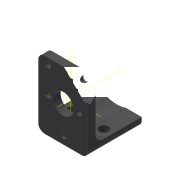
# Autodesk Inventor part: empty
Saved by Autodesk Inventor 2014 (Build 180170000, 170)
## iProperties
Created: 2015-04-13
Part Number: empty
Material: Generic
Document SubType Name: Modeling
Designer: Martin
Density: 1 g/cm^3
Appearance: Default
Author: Martin
Autodesk Inventor part; units mm, degrees
ref_plane "YZ Plane" through (0, 0, 0) normal (1, 0, 0) x (0, 1, 0)
ref_plane "XZ Plane" through (0, 0, 0) normal (0, 1, 0) x (-1, 0, 0)
ref_plane "XY Plane" through (0, 0, 0) normal (0, 0, 1) x (1, 0, 0)
sketch "sk_main" plane through (0, 0, 0) normal (1, 0, 0) x (0, 1, 0)
  line L0 (-8, 0) -> (30.5, 0) projected
  line L1 (0, -15.9) -> (0, 14.9) projected
  line L2 (25, -7.5) -> (0, -7.5)
  line L3 (0, -7.5) -> (0, 9)
  line L4 (25, -11.5) -> (-2.5, -11.5)
  line L5 (-2.5, -11.5) -> (-2.5, 10.5)
  line L6 (0, 10.5) -> (0, -11.5)
  line L7 (25, -7.5) -> (25, -11.5)
  line L8 (-2.5, 10.5) -> (0, 10.5)
  point P0 (0, 0)
  dimension "d5" = 2.5
  dimension "d35" = 25
  dimension "d37" = 4
  dimension "d38" = 18
  dimension "d58" = 10.5
  constraints: 14 end point, 4 perpendicular, 3 point on line, 1 collinear, 1 horizontal, 1 parallel
  measures "d5" distance between parallel lines of L3 L5
  measures "d35" distance of L2.start L2.end
  measures "d37" distance of L2.start L4.start
  measures "d38" distance between parallel lines of L2 L8
  measures "d58" distance between parallel lines of L8 L0
extrude "ext_main_back" [suppressed]
extrude "ext_main_front" add sketch "sk_main" along normal mid plane 12.15 contours L5 L8 L1 L0 | L0 L1 L4 L5
sketch "sk_front" plane through (0, 0, 0) normal (0, 1, 0) x (-1, 0, 0)
  line L0 (0, -22.55) -> (0, 16.3) projected
  line L1 (12.1092, 0) -> (-12.1092, 0) projected
  circle A0 centre (0, 0) radius 3.4
  circle A1 centre (5.075, 0) radius 1
  circle A2 centre (-5.075, 0) radius 1
  circle A3 centre (0, 0) radius 8 construction
  circle A4 centre (0, -9) radius 8 construction
  circle A5 centre (0, -9) radius 1
  line L2 (8.6494, -4.5) -> (-8.6494, -4.5) construction
  line L3 (-6.075, 10.5) -> (-6.075, -11.5) projected
  line L4 (6.075, -11.5) -> (6.075, 10.5) projected
  line L5 (6.075, -11.5) -> (-6.075, -11.5) projected
  circle A6 centre (-5, 8.5) radius 1
  circle A7 centre (-5, 8.5) radius 2.25 construction
  line L6 (-5, 8.5) -> (5, 8.5) construction
  circle A8 centre (5, 8.5) radius 2.25 construction
  circle A9 centre (5, 8.5) radius 1
  line L7 (6.075, 10.5) -> (6.075, -11.5)
  line L8 (6.075, -11.5) -> (8.075, -11.5)
  line L9 (8.075, -11.5) -> (8.075, 10.5)
  line L10 (8.075, 10.5) -> (6.075, 10.5)
  line L11 (-6.075, -11.5) -> (-6.075, 10.5)
  line L12 (-6.075, 10.5) -> (-8.075, 10.5)
  line L13 (-8.075, 10.5) -> (-8.075, -11.5)
  line L14 (-8.075, -11.5) -> (-6.075, -11.5)
  point P0 (0, 8.5)
  dimension "d11" = 6.8
  dimension "d12" = 2
  dimension "d13" = 10.15
  dimension "d14" = 16
  dimension "d15" = 16
  dimension "d16" = 9
  dimension "d17" = 2
  dimension "d27" = 2
  dimension "d28" = 4.5
  dimension "d30" = 10
  dimension "d31" = 8.5
  dimension "d39" = 2
  constraints: 20 end point, 10 centre point, 7 parallel, 6 coincident, 5 perpendicular, 5 point on line, 3 equal radius, 2 symmetric about line, 1 collinear, 1 midpoint
  measures "d11" diameter of A0
  measures "d12" diameter of A2
  measures "d13" distance of A2.centre A1.centre
  measures "d14" diameter of A3
  measures "d15" diameter of A4
  measures "d16" distance of A4.centre point (0, 0)
  measures "d17" diameter of A5
  measures "d27" diameter of A6
  measures "d28" diameter of A7
  measures "d30" distance of L6.start L6.end
  measures "d31" distance between parallel lines of L1 L6
  measures "d39" distance of L9.end L4.end
extrude "ext_front_tabs" add sketch "sk_front" against normal up to surface (2.5 mm away) contours L4 L1 L9 L8 | L14 L13 L1 L3 | L4 L10 L9 L1 | L1 L13 L12 L3
extrude "ext_cut_holesfront" cut sketch "sk_front" against normal through all contours A5 L0 | L0 A5 | A1 L1 | L1 A1 | A2 L1 | L1 A2 | A0 L1 L0 | L0 L1 A0 | L1 A0 L0 | L0 A0 L1 | A6 | A9
fillet "Fillet5" radius 2 4 edges at (-8.075, -1.25, -11.5) (8.075, -1.25, -11.5) (8.075, -1.25, 10.5) (-8.075, -1.25, 10.5)
sketch "Sketch7" plane through (8.075, 0, 8.5) normal (0, 1, 0) x (1, 0, 0)
  line L0 (0, 0) -> (0, 18) projected
  arc A0 (0, 18) -> (-2, 20) centre (-2, 18) ccw projected
  line L1 (-14.15, 20) -> (-2, 20) projected
  arc A1 (-14.15, 20) -> (-16.15, 18) centre (-14.15, 18) ccw projected
  line L2 (-16.15, 18) -> (-16.15, 0) projected
  circle A2 centre (-8.075, 8.5) radius 3.4 projected
  circle A3 centre (-8.075, 8.5) radius 9
  line L3 (-11.033, 17) -> (-16.15, 17)
  line L4 (-5.117, 17) -> (0, 17)
  line L5 (-2, -2) -> (-14.15, -2) projected
  line L6 (-16.15, 17) -> (-16.15, 21)
  line L7 (-16.15, 21) -> (0, 21)
  line L8 (0, 21) -> (0, 17)
  dimension "d45" = 18
  dimension "d46" = 3
  dimension "d57" = 1
  constraints: 10 end point, 3 perpendicular, 2 equal length, 2 point on circle, 2 point on line, 1 centre point, 1 coincident, 1 collinear
  measures "d45" diameter of A3
  measures "d46" distance between parallel lines of L1 L3
  measures "d57" distance between parallel lines of L1 L7
extrude "ext_backtab" add sketch "Sketch7" along normal blind 15 contours L4 A3 L3 L2 A1 L1 A0 L0
sketch "Sketch8" plane through (6.075, -2.5, -11.5) normal (0, 0, -1) x (-1, 0, 0)
  line L0 (12.15, 0) -> (0, 0) projected
  line L1 (0, 17.5) -> (12.15, 17.5) projected
  line L2 (6.075, 0) -> (6.075, 17.5)
  circle A0 centre (0.825, 8) radius 1.5
  circle A1 centre (11.325, 8) radius 1.5
  line L3 (0.825, 8) -> (11.325, 8) construction
  point P0 (6.075, 2.5)
  dimension "d49" = 3
  dimension "d50" = 10.5
  dimension "d56" = 8
  constraints: 4 end point, 2 centre point, 2 midpoint, 1 other
  measures "d49" diameter of A1
  measures "d50" distance of L3.start L3.end
  measures "d56" distance between parallel lines of L0 L3
extrude "ext_cut_mountholes" cut sketch "Sketch8" against normal up to next
fillet "Fillet6" radius 2.5 2 edges at (5.5165, 0, -8.5) (-5.5165, 0, -8.5)
extrude "ext_dowelfill" add sketch "sk_front" against normal blind 1.7 contours A5 L0 | L0 A5
equation "\"d12\" = screw_m2_bore_selfthreading"
equation "\"d17\" = screw_m2_bore_selfthreading"
equation "\"d27\" = screw_m2_bore_selfthreading"
equation "\"d28\" = screw_m2_head_maxsize"
equation "\"d49\" = screw_m3_bore_selfthreading"
equation "\"screw_m2_bore_selfthreading\" = 2"
equation "\"screw_m2_head_maxsize\" = 4.5"
equation "\"screw_m3_bore_selfthreading\" = 3"
body "Solid1"
